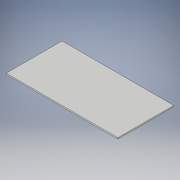
# Autodesk Inventor part: mat
Saved by Autodesk Inventor 2019.4 (Build 234330000, 330)
## iProperties
Created: 2020-11-10
Part Number: mat
Material: 一般
Document SubType Name: Modeling
Designer: kawap
Density: 1 g/cm^3
Appearance: 既定
Author: kawap
Autodesk Inventor part; units mm, degrees
ref_plane "YZ Plane" through (0, 0, 0) normal (1, 0, 0) x (0, 1, 0)
ref_plane "XZ Plane" through (0, 0, 0) normal (0, 1, 0) x (-1, 0, 0)
ref_plane "XY Plane" through (0, 0, 0) normal (0, 0, 1) x (1, 0, 0)
sketch "スケッチ1" plane through (0, 0, 0) normal (0, 1, 0) x (-1, 0, 0)
  line L0 (90, -45) -> (-90, -45)
  line L1 (-90, -45) -> (-90, 45)
  line L2 (-90, 45) -> (90, 45)
  line L3 (90, 45) -> (90, -45)
  line L4 (90, -45) -> (-90, 45) construction
  line L5 (-90, -45) -> (90, 45) construction
  point P0 (0, 0)
  dimension "d0" = 180
  dimension "d1" = 90
  constraints: 12 end point, 2 midpoint, 2 parallel, 1 horizontal, 1 perpendicular
  measures "d0" distance of L1.end L2.end
  measures "d1" distance of L0.end L1.end
extrude "押し出し1" add sketch "スケッチ1" along normal blind 2
